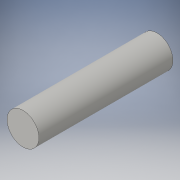
# Autodesk Inventor part: rod
Saved by Autodesk Inventor 2016 (Build 200138000, 138)
## iProperties
Created: 2017-06-27
Part Number: rod
Material: Generic
Document SubType Name: Modeling
Designer: M228854
Density: 1 g/cm^3
Appearance: Default
Author: M228854
Autodesk Inventor part; units mm, degrees
ref_plane "YZ Plane" through (0, 0, 0) normal (1, 0, 0) x (0, 1, 0)
ref_plane "XZ Plane" through (0, 0, 0) normal (0, 1, 0) x (-1, 0, 0)
ref_plane "XY Plane" through (0, 0, 0) normal (0, 0, 1) x (1, 0, 0)
sketch "Sketch1" plane through (0, 0, 0) normal (0, 0, 1) x (1, 0, 0)
  circle A0 centre (0, 0) radius 9.9
  dimension "d0" = 19.8
  constraints: 1 centre point, 1 coincident
  measures "d0" diameter of A0
extrude "Extrusion1" add sketch "Sketch1" along normal blind 83.3
body "Solid1"
